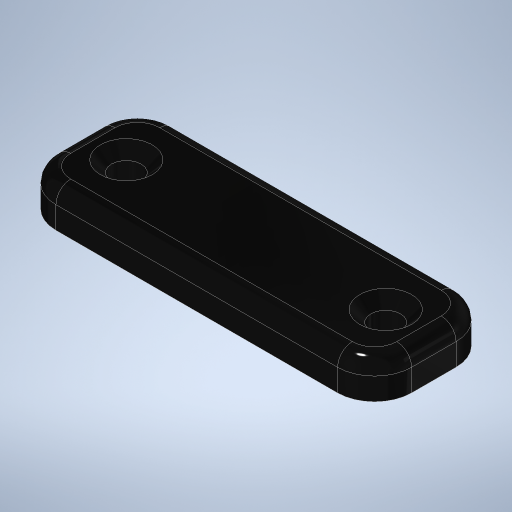
# Autodesk Inventor part: Support 48x16
Saved by Autodesk Inventor 2024 (Build 280153000, 153)
## iProperties
Category: Supports and legs
Created: 2007-05-26
Part Number: Support 48x16
Material: ABS Plastic
Document SubType Name: Modeling
Designer: G.K.
Description: Support 48 x 16
Authority: Design by UAB Čeli APS
Density: 1.06 g/cm^3
Appearance: Glossy - Black
Author: G.K.
Title: Simple support 48 x 16
Subject: Support
Keywords: support, 48x16, black, plastic
Comments: support, 48x16, black, plastic
Revision Number: 1
Autodesk Inventor part; units mm, degrees
ref_plane "YZ Plane" through (0, 0, 0) normal (1, 0, 0) x (0, 1, 0)
ref_plane "XZ Plane" through (0, 0, 0) normal (0, 1, 0) x (-1, 0, 0)
ref_plane "XY Plane" through (0, 0, 0) normal (0, 0, 1) x (1, 0, 0)
sketch "Sketch1" plane through (0, 0, 0) normal (0, 0, 1) x (1, 0, 0)
  line L0 (24, -8) -> (-24, -8)
  line L1 (-24, -8) -> (-24, 8)
  line L2 (-24, 8) -> (24, 8)
  line L3 (24, 8) -> (24, -8)
  point P0 (0, 0)
  point P1 (-24, 0)
  point P2 (0, 8)
  dimension "d0" = 48
  dimension "d1" = 16
  constraints: 8 end point, 2 midpoint, 2 parallel, 1 horizontal, 1 horizontal alignment, 1 perpendicular, 1 vertical alignment
  measures "d0" distance of L0.start L0.end
  measures "d1" distance of L2.end L0.start
extrude "Extrusion1" add sketch "Sketch1" along normal blind 5
fillet "Fillet1" radius 5 4 edges at (-24, -8, 2.5) (-24, 8, 2.5) (24, -8, 2.5) (24, 8, 2.5)
fillet "Fillet2" radius 2 8 edges at (0, -8, 5) (-22.5355, -6.5355, 5) (-24, 0, 5) (-22.5355, 6.5355, 5) (0, 8, 5) (22.5355, 6.5355, 5) (24, 0, 5) (22.5355, -6.5355, 5)
sketch "Sketch2" plane through (0, 0, 5) normal (0, 0, 1) x (1, 0, 0)
  line L0 (19, -6) -> (-19, -6) projected
  line L1 (22, 3) -> (22, -3) projected
  line L2 (-19, 6) -> (19, 6) projected
  line L3 (-22, -3) -> (-22, 3) projected
  line L4 (-22, 0) -> (22, 0) construction
  line L5 (0, 6) -> (0, -6) construction
  point P0 (0, 0)
  point P1 (-17.5, 0)
  point P2 (17.5, 0)
  dimension "d6" = 35
  constraints: 4 end point, 4 midpoint, 2 point on line, 1 symmetric about line
  measures "d6" distance of point (17.5, 0) point (-17.5, 0)
hole "Hole1" at (-17.5, 0, 5) at (17.5, 0, 5) direction (0, 0, -1) diameter 4 end through all countersink diameter 7 countersink angle 90
body "Solid1"
